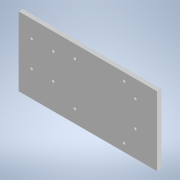
# Autodesk Inventor part: lidar_plate
Saved by Autodesk Inventor 2021 (Build 250183000, 183)
## iProperties
Created: 2020-10-27
Part Number: lidar_plate
Material: Generic
Document SubType Name: Modeling
Designer: Mateusz
Density: 1 g/cm^3
Appearance: Default
Author: Mateusz
Autodesk Inventor part; units mm, degrees
ref_plane "YZ Plane" through (0, 0, 0) normal (1, 0, 0) x (0, 1, 0)
ref_plane "XZ Plane" through (0, 0, 0) normal (0, 1, 0) x (-1, 0, 0)
ref_plane "XY Plane" through (0, 0, 0) normal (0, 0, 1) x (1, 0, 0)
sketch "Sketch2" plane through (0, 0, 0) normal (0, 0, 1) x (1, 0, 0)
  line L0 (40, -40) -> (-70, -40)
  line L1 (-70, -40) -> (-70, 40)
  line L2 (-70, 40) -> (40, 40)
  circle A0 centre (-35, -25) radius 1 projected
  circle A1 centre (-35, -25) radius 1.45
  circle A2 centre (22, -31) radius 1 projected
  circle A3 centre (22, -31) radius 1.45
  circle A4 centre (22, 31) radius 1 projected
  circle A5 centre (22, 31) radius 1.45
  circle A6 centre (-35, 25) radius 1 projected
  circle A7 centre (-35, 25) radius 1.45
  line L3 (59.9998, -0.0003) -> (34.9998, -0.0003)
  line L4 (34.9998, -0.0003) -> (34.9998, -10.1033)
  line L5 (34.9998, -0.0003) -> (34.9998, 19.8967)
  circle A8 centre (34.9998, -10.1033) radius 1.45
  circle A9 centre (34.9998, 19.8967) radius 1.45
  line L6 (-60, 0) -> (-60, -10.103)
  line L7 (-60, -10.103) -> (-60, 0)
  line L8 (-60, 0) -> (-60, 19.897)
  circle A10 centre (-60, 19.897) radius 1.45
  circle A11 centre (-60, -10.103) radius 1.45
  line L9 (40, -40) -> (60, -40)
  line L10 (60, -40) -> (60, 40)
  line L11 (60, 40) -> (40, 40)
  line L12 (60, -40) -> (60, 0)
  line L13 (-70, 0) -> (-60, 0)
  point P0 (0, 0)
  dimension "d1" = 44.721
  dimension "d2" = 110
  dimension "d3" = 80
  dimension "d4" = 2.9
  dimension "d5" = 2.9
  dimension "d6" = 2.9
  dimension "d7" = 2.9
  dimension "d8" = 25
  dimension "d9" = 10.103
  dimension "d11" = 19.897
  dimension "d12" = 2.9
  dimension "d13" = 2.9
  dimension "d19" = 2.9
  dimension "d20" = 2.9
  dimension "d21" = 20
  dimension "d22" = 10
  constraints: 28 end point, 8 centre point, 8 coincident, 4 perpendicular, 2 collinear, 2 horizontal, 2 vertical, 1 midpoint, 1 point on line
  measures "d1" distance of L3.start L0.start
  measures "d2" distance of L0.start L0.end
  measures "d3" distance of L0.end L1.end
  measures "d4" diameter of A1
  measures "d5" diameter of A3
  measures "d6" diameter of A5
  measures "d7" diameter of A7
  measures "d8" distance of L3.start L3.end
  measures "d9" distance of L3.end L4.end
  measures "d11" distance of L3.end L5.end
  measures "d12" diameter of A8
  measures "d13" diameter of A9
  measures "d19" diameter of A10
  measures "d20" diameter of A11
  measures "d21" distance of L0.start L9.end
  measures "d22" distance of L13.start L13.end
extrude "Extrusion1" add sketch "Sketch2" along normal blind 5 contours L0 L1 L2 L11 L10 L9
sketch "Sketch3" plane through (0, 0, 0) normal (0, 0, -1) x (-1, 0, 0)
  line L0 (70, 40) -> (70, -40) projected
  line L1 (70, 40) -> (100, 40)
  line L2 (100, 40) -> (100, -40)
  line L3 (100, -40) -> (70, -40)
  line L4 (70, -40) -> (70, 40)
  circle A0 centre (85, 19.9314) radius 1.45
  circle A1 centre (85, -10.0686) radius 1.45
  point P0 (0, 0)
  dimension "d23" = 30
  dimension "d25" = 2.9
  dimension "d26" = 2.9
  constraints: 8 end point, 2 centre point, 2 perpendicular, 1 collinear, 1 horizontal
  measures "d23" distance of L0.start L1.end
  measures "d25" diameter of A0
  measures "d26" diameter of A1
extrude "Extrusion2" add sketch "Sketch3" against normal up to surface (5 mm away)
body "Solid2"
